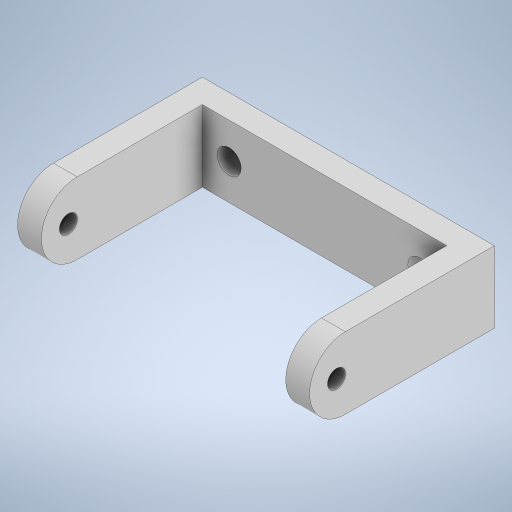
# Autodesk Inventor part: Zebatka holderv2
Saved by Autodesk Inventor 2024 (Build 280153000, 153)
## iProperties
Created: 2025-05-18
Part Number: Zebatka holderv2
Material: Ogólny
Document SubType Name: Modeling
Designer: Victoria
Density: 1 g/cm^3
Appearance: Domyślna
Author: Victoria
Autodesk Inventor part; units mm, degrees
ref_plane "YZ Plane" through (0, 0, 0) normal (1, 0, 0) x (0, 1, 0)
ref_plane "XZ Plane" through (0, 0, 0) normal (0, 1, 0) x (-1, 0, 0)
ref_plane "XY Plane" through (0, 0, 0) normal (0, 0, 1) x (1, 0, 0)
sketch "Szkic1" plane through (0, 0, 0) normal (0, 0, 1) x (1, 0, 0)
  line L0 (0, 0) -> (-32, 0)
  circle A0 centre (-32, 0) radius 2
  circle A1 centre (0, 0) radius 2
  line L1 (-40.5, -6) -> (8.5, -6)
  line L2 (8.5, -6) -> (8.5, 6)
  line L3 (8.5, 6) -> (-40.5, 6)
  line L4 (-40.5, 6) -> (-40.5, -6)
  line L5 (-40.5, -6) -> (8.5, 6) construction
  line L6 (8.5, -6) -> (-40.5, 6) construction
  point P0 (-16, 0)
  dimension "d2" = 32
  dimension "d3" = 4
  dimension "d4" = 4
  dimension "d5" = 49
  dimension "d6" = 12
  constraints: 14 end point, 3 midpoint, 2 centre point, 2 coincident, 2 horizontal, 2 parallel, 1 perpendicular
  measures "d2" distance of L0.start L0.end
  measures "d3" diameter of A0
  measures "d4" diameter of A1
  measures "d5" distance of L3.end L2.end
  measures "d6" distance of L2.end L1.end
extrude "Wyciągnięcie proste1" add sketch "Szkic1" along normal blind 5
sketch "Szkic2" plane through (0, 0, 5) normal (0, 0, 1) x (1, 0, 0)
  line L0 (8.5, -6) -> (8.5, 6) projected
  line L1 (-40.5, -6) -> (8.5, -6) projected
  line L2 (8.5, 6) -> (4.5, 6)
  line L3 (4.5, 6) -> (4.5, -6)
  line L4 (4.5, -6) -> (8.5, -6)
  line L5 (8.5, -6) -> (8.5, 6)
  line L6 (-40.5, 6) -> (-36.5, 6)
  line L7 (-36.5, 6) -> (-36.5, -6)
  line L8 (-36.5, -6) -> (-40.5, -6)
  line L9 (-40.5, -6) -> (-40.5, 6)
  dimension "d12" = 4
  dimension "d13" = 4
  constraints: 16 end point, 4 parallel, 2 horizontal, 2 perpendicular, 2 point on line
  measures "d12" distance of L4.end L3.end
  measures "d13" distance of L7.end L8.end
extrude "Wyciągnięcie proste2" add sketch "Szkic2" along normal blind 26
fillet "Zaokrąglenie1" radius 6 4 edges at (-38.5, 6, 31) (-38.5, -6, 31) (6.5, 6, 31) (6.5, -6, 31)
sketch "Szkic3" plane through (-36.5, -6, 5) normal (1, 0, 0) x (0, 0, -1)
  line L0 (0, 5.9057) -> (-21.5, 5.9057)
  circle A0 centre (-21.5, 5.9057) radius 1.5
  point P0 (5, 6)
  dimension "d15" = 21.5
  dimension "d16" = 3
  constraints: 2 end point, 1 centre point, 1 coincident, 1 horizontal
  measures "d15" distance of L0.start L0.end
  measures "d16" diameter of A0
extrude "Wyciągnięcie proste3" cut sketch "Szkic3" along normal mid plane 100
sketch "Szkic4" plane through (0, 0, 5) normal (0, 0, 1) x (1, 0, 0)
  circle A0 centre (0, 0) radius 2 projected
  circle A1 centre (-32, 0) radius 2 projected
  line L0 (4.5, -6) -> (4.5, 6) projected
  line L1 (4.5, 6) -> (-36.5, 6) projected
  line L2 (-36.5, 6) -> (-36.5, -6) projected
  line L3 (-36.5, -6) -> (4.5, -6) projected
extrude "Wyciągnięcie proste4" cut sketch "Szkic4" against normal blind 1 contours A0 | A1 | L3 L2 L1 L0
